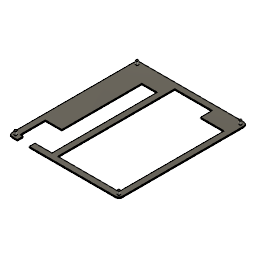
EasySplit-Right-Top (Autodesk Fusion 360 design; units mm, degrees)
part number: 2026-04-16-19-10-06-869
Autodesk Fusion 360 part; units mm, degrees
sketch "Sketch1" plane through (0, 0, 0) normal (0, 0, 1) x (1, 0, 0)
  line L0 (167.6875, -193.6438) -> (-20, -193.6438)
  line L1 (-10, 15) -> (157.6875, 15)
  line L2 (-20, -193.6438) -> (-20, 25)
  line L3 (167.6875, 25) -> (167.6875, -193.6438)
  line L4 (-10, -183.6438) -> (-10, 15)
  line L5 (157.6875, 15) -> (157.6875, -183.6438)
  line L6 (157.6875, -183.6438) -> (-10, -183.6438)
  line L7 (-20, 25) -> (167.6875, 25)
  line L8 (15, -183.6438) -> (-5, -183.6438)
  line L9 (-5, -183.6438) -> (-5, -193.6438)
  line L10 (-5, -193.6438) -> (15, -193.6438)
  line L11 (15, -193.6438) -> (15, -183.6438)
  line L12 (-10, 15) -> (18, 15)
  line L13 (18, 15) -> (18, -141)
  line L14 (18, -141) -> (-10, -141)
  line L15 (-10, -141) -> (-10, 15)
  line L16 (44, 15) -> (54, 15)
  line L17 (54, 15) -> (54, -185)
  line L18 (54, -185) -> (44, -185)
  line L19 (44, -185) -> (44, 15)
  line L20 (157.6875, -183.6438) -> (121.6875, -183.6438)
  line L21 (121.6875, -183.6438) -> (121.6875, -148.1438)
  line L22 (121.6875, -148.1438) -> (157.6875, -148.1438)
  line L23 (157.6875, -148.1438) -> (157.6875, -183.6438)
  line L24 (18, -141) -> (44, -141)
  line L25 (14, -141) -> (18, -141)
  line L26 (18, 15) -> (44, 15)
  line L27 (44, 15) -> (44, -5)
  line L28 (44, -5) -> (18, -5)
  line L29 (18, -5) -> (18, 15)
  line L30 (157.6875, 15) -> (117.6875, 15)
  line L31 (117.6875, 15) -> (117.6875, -5)
  line L32 (117.6875, -5) -> (157.6875, -5)
  line L33 (157.6875, -5) -> (157.6875, 15)
  dimension "d3" = 167.6875
  dimension "d4" = 198.6438
  dimension "d5" = 187.6875
  dimension "d6" = 218.6438
  dimension "d7" = 10
  dimension "d8" = 10
  dimension "d19" = 20
  dimension "d20" = 15
  dimension "d21" = 28
  dimension "d22" = 156
  dimension "d23" = 10
  dimension "d24" = 200
  dimension "d25" = 26
  dimension "d26" = 36
  dimension "d27" = 35.5
  dimension "d29" = 10
  dimension "d30" = 20
  dimension "d31" = 40
  dimension "d32" = 20
  constraint horizontal L1
  constraint vertical L5
  constraint horizontal L6
  constraint vertical L4
  constraint horizontal L7
  constraint vertical L3
  constraint horizontal L0
  constraint vertical L2
  constraint horizontal L8
  constraint vertical L9
  constraint horizontal L10
  constraint vertical L11
  constraint coincident L6 L8.start
  constraint horizontal L12
  constraint vertical L13
  constraint horizontal L14
  constraint vertical L15
  constraint horizontal L16
  constraint vertical L17
  constraint horizontal L18
  constraint vertical L19
  constraint coincident L1 L16.start
  constraint horizontal L20
  constraint vertical L21
  constraint horizontal L22
  constraint vertical L23
  constraint horizontal L24
  constraint horizontal L25
  constraint coincident L14 L25.start
  constraint horizontal L26
  constraint vertical L27
  constraint horizontal L28
  constraint vertical L29
  constraint horizontal L30
  constraint vertical L31
  constraint horizontal L32
  constraint vertical L33
  measures "d3" distance of L1.start L1.end
  measures "d4" distance of L1.start L4.start
  measures "d5" distance of L2.end L3.start
  measures "d6" distance of L2.end L0.end
  measures "d7" distance of L1 L7
  measures "d8" distance of L2 L4
  measures "d19" distance of L8.start L8.end
  measures "d20" distance of L2 L9
  measures "d21" distance of L1.start L12.end
  measures "d22" distance of L1.start L14.end
  measures "d23" distance of L16.start L16.end
  measures "d24" distance of L16.start L18.end
  measures "d25" distance of L13 L19
  measures "d26" distance of L5.end L20.end
  measures "d27" distance of L5.end L22.end
  measures "d29" distance of L8.start L10.end
  measures "d30" distance of L12.end L28.end
  measures "d31" distance of L1.end L30.end
  measures "d32" distance of L1.end L32.end
extrude "Extrude1" add sketch "Sketch1" along normal blind 2 contours L0 L1 L2 L3 L4 L5 L6 L7 L9 L11 L12 L15 L16 L17 L18 L19 L20 L23 L26 L30 L33 | L1 L6 L16 L17 L19 L27 | L6 L17 L18 L19 | L1 L4 L12 L13 L14 L15 L25 L29 | L1 L13 L19 L26 L27 L28 L29 | L1 L5 L30 L31 L32 L33
fillet "Fillet1" radius 6 1 edges at (167.6875, -193.6438, 1)
fillet "Fillet2" radius 6 1 edges at (167.6875, 25, 1)
fillet "Fillet3" radius 6 1 edges at (-20, 25, 1)
fillet "Fillet4" radius 6 1 edges at (-20, -193.6438, 1)
move_face "MoveFace1" to x (-1, 0, 0) y (0, 1, 0) z (0, 0, -1) at (108, 0, 4) 1 faces at (-4, -42.3333, 2)
sketch "Sketch2" plane through (0, 0, 2) normal (0, 0, 1) x (-1, 0, 0)
  arc A0 (20, 187.6438) -> (14, 193.6438) centre (14, 187.6438) ccw
  line L0 (14, 193.6438) -> (5, 193.6438)
  line L1 (5, 193.6438) -> (5, 183.6438)
  line L2 (5, 183.6438) -> (10, 183.6438)
  line L3 (10, 183.6438) -> (10, 141)
  line L4 (10, 141) -> (-18, 141)
  line L5 (-18, 141) -> (-18, 5)
  line L6 (-18, 5) -> (-44, 5)
  line L7 (-44, 5) -> (-44, 183.6438)
  line L8 (-44, 183.6438) -> (-15, 183.6438)
  line L9 (-15, 183.6438) -> (-15, 193.6438)
  line L10 (-15, 193.6438) -> (-161.6875, 193.6438)
  arc A1 (-161.6875, 193.6438) -> (-167.6875, 187.6438) centre (-161.6875, 187.6438) ccw
  line L11 (-167.6875, 187.6438) -> (-167.6875, -19)
  arc A2 (-167.6875, -19) -> (-161.6875, -25) centre (-161.6875, -19) ccw
  line L12 (-161.6875, -25) -> (14, -25)
  arc A3 (14, -25) -> (20, -19) centre (14, -19) ccw
  line L13 (20, -19) -> (20, 187.6438)
  line L14 (-54, 183.6438) -> (-54, -15)
  line L15 (-54, -15) -> (-117.6875, -15)
  line L16 (-117.6875, -15) -> (-117.6875, 5)
  line L17 (-117.6875, 5) -> (-157.6875, 5)
  line L18 (-157.6875, 5) -> (-157.6875, 183.6438)
  line L19 (-157.6875, 183.6438) -> (-54, 183.6438)
  circle A4 centre (14, -19) radius 2.1
  circle A5 centre (-161.6875, -19) radius 2.1
  circle A6 centre (-161.6875, 187.6438) radius 2.1
  circle A7 centre (14, 187.6438) radius 2.1
  dimension "d33" = 4.2
  dimension "d34" = 4.2
  dimension "d35" = 4.2
  dimension "d36" = 4.2
  dimension "d37" = 6
  dimension "d38" = 6
  dimension "d39" = 6
  dimension "d40" = 6
  dimension "d41" = 6
  dimension "d42" = 6
  dimension "d43" = 6
  dimension "d44" = 6
  measures "d33" diameter of A4
  measures "d34" diameter of A5
  measures "d35" diameter of A6
  measures "d36" diameter of A7
  measures "d37" distance of L0 A0.centre
  measures "d38" distance of L13 A0.centre
  measures "d39" distance of L13 A3.centre
  measures "d40" distance of L12 A3.centre
  measures "d41" distance of L11 A2.centre
  measures "d42" distance of L12 A2.centre
  measures "d43" distance of L10 A1.centre
  measures "d44" distance of L11 A1.centre
extrude "Extrude2" add sketch "Sketch2" along normal blind 6 contours A4 | A5 | A6 | A7
